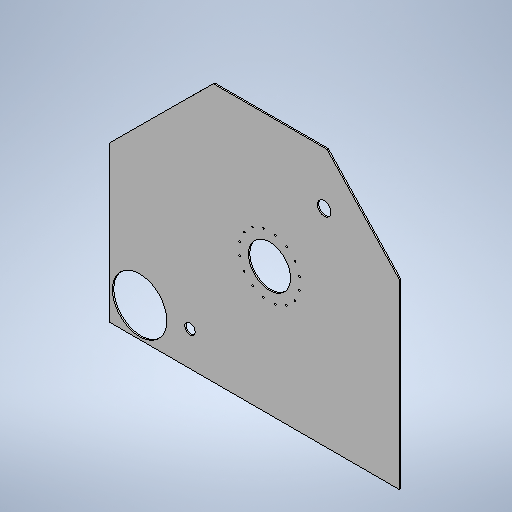
# Autodesk Inventor part: Left wall v2.0
Saved by Autodesk Inventor 2026.2 (Build 302298010, 298A)
## iProperties
Created: 2023-08-31
Part Number: Left wall v2.0
Material: Generic
Document SubType Name: Sheet Metal
Designer: admin
Density: 1 g/cm^3
Appearance: Default
Flat Pattern Width: 191 cm
Flat Pattern Length: 214 cm
Flat Pattern Area: 40874 cm^2
Sheet Metal Rule: Default
Sheet Metal Width: 1910,000 mm
Sheet Metal Length: 2140,000 mm
Sheet Metal Area: 4087400,000 mm^2
Stock Number: ДМФ 013 Стенка Нос
Author: admin
Autodesk Inventor part; units mm, degrees
ref_plane "YZ Plane" through (0, 0, 0) normal (1, 0, 0) x (0, 1, 0)
ref_plane "XZ Plane" through (0, 0, 0) normal (0, 1, 0) x (-1, 0, 0)
ref_plane "XY Plane" through (0, 0, 0) normal (0, 0, 1) x (1, 0, 0)
sketch "Sketch1" plane through (0, 0, 0) normal (0, 0, 1) x (1, 0, 0)
  line L0 (0, 0) -> (0, 1910) construction
  line L1 (424.5155, 1910) -> (-415.4845, 1910)
  line L2 (-415.4845, 1910) -> (-1180, 1150)
  line L3 (-1180, 0) -> (-1180, 1150)
  line L4 (960, 0) -> (960, 1342.8524)
  line L5 (424.5155, 1910) -> (960, 1342.8524)
  circle A0 centre (0, 950) radius 195 construction
  line L6 (960, 0) -> (-1180, 0)
  circle A1 centre (-960, 220) radius 200.5
  circle A2 centre (-588, 255) radius 38
  circle A3 centre (0, 950) radius 155
  circle A4 centre (0, 950) radius 700 construction
  line L7 (404.31, 1277) -> (404.31, 1910) construction
  circle A5 centre (404.31, 1521.431) radius 50
  point P0 (0, 955)
  dimension "d69" = 1400
  dimension "d1" = 840
  dimension "d3" = 1150
  dimension "d11" = 390
  dimension "d12" = 1180
  dimension "d13" = 950
  dimension "d14" = 76
  dimension "d15" = 1910
  dimension "d16" = 255
  dimension "d17" = 220
  dimension "d18" = 401
  dimension "d19" = 220
  dimension "d33" = 2140
  dimension "d45" = 310
  dimension "d49" = 372
  dimension "d51" = 780
  dimension "d52" = 1078
  dimension "d70" = 1584.31
  dimension "d71" = 100
  constraints: 16 end point, 5 centre point, 5 point on line, 3 vertical, 2 horizontal, 1 coincident, 1 midpoint, 1 perpendicular, 3 other
  measures "d1" distance of L1.start L1.end
  measures "d3" distance of L3.start L2.end
  measures "d11" diameter of A0
  measures "d12" distance from line of L3 A0.centre
  measures "d13" distance from line of L6 A0.centre
  measures "d14" diameter of A2
  measures "d15" vertical distance of L3.start L1.end
  measures "d16" distance from line of A2.centre L6
  measures "d17" distance from line of L3 A1.centre
  measures "d18" diameter of A1
  measures "d19" distance from line of A1.centre L6
  measures "d33" distance of L4.start L3.start
  measures "d45" diameter of A3
  measures "d49" horizontal distance of A1.centre A2.centre
  measures "d51" distance of L1.start L4.end
  measures "d52" distance of L1.end L2.end
  measures "d70" distance between parallel lines of L3 L7
  measures "d71" diameter of A5
extrude "Extrusion1" add sketch "Sketch1" along normal blind 10
sketch "Sketch4" plane through (0, 0, 0) normal (0, 0, -1) x (-1, 0, 0)
  circle A0 centre (960, 220) radius 200.5 projected
  circle A1 centre (588, 255) radius 38 projected
  line L0 (-960, 1342.8524) -> (-424.5155, 1910) projected
  line L1 (-960, 0) -> (-960, 1342.8524) projected
  line L2 (1180, 0) -> (-960, 0) projected
  line L3 (1180, 1150) -> (1180, 0) projected
  line L4 (415.4845, 1910) -> (1180, 1150) projected
  line L5 (-424.5155, 1910) -> (415.4845, 1910) projected
  circle A2 centre (0, 950) radius 155 projected
  circle A3 centre (0, 950) radius 210
  circle A4 centre (0, 950) radius 250
  point P0 (0, 0)
  dimension "d53" = 500
  dimension "d54" = 420
  constraints: 2 centre point, 1 coincident
  measures "d53" diameter of A4
  measures "d54" diameter of A3
extrude "Extrusion4" add sketch "Sketch4" along normal blind 10 contours A4
sketch "Sketch5" plane through (0, 0, 0) normal (0, 0, -1) x (-1, 0, 0)
  circle A0 centre (0, 950) radius 155 projected
  circle A1 centre (0, 950) radius 225 construction
  point P0 (0, 0)
  point P1 (43.4498, 1170.7648)
  dimension "d57" = 450
  constraints: 1 centre point, 1 coincident, 3 other
hole "Hole1" at (-43.4498, 1170.7648, 0) direction (0, 0, 1) diameter 12 end through all both
pattern_circular "Circular Pattern2" count 16 over 360 about axis through (0, 950, 0) along (0, 0, 1) of "Hole1"
equation "\"d17\" = d19"
body "Solid1"
